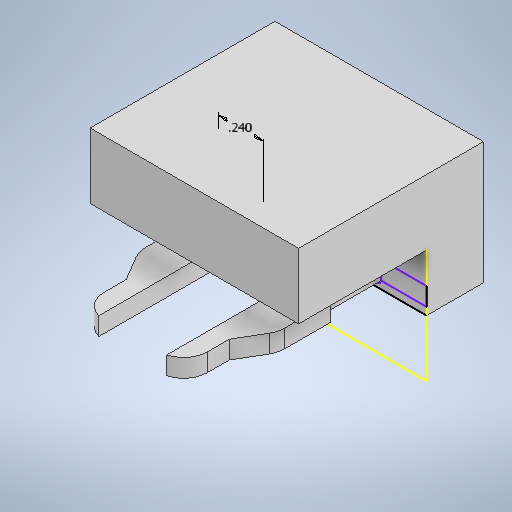
# Autodesk Inventor part: Attachment1
Saved by Autodesk Inventor 2025 (Build 290162010, 162A)
## iProperties
Created: 2026-02-26
Part Number: Attachment1
Material: Generic
Document SubType Name: Modeling
Designer: 925699
Density: 1 g/cm^3
Appearance: Default
Author: 925699
Autodesk Inventor part; units mm, degrees
ref_plane "YZ Plane" through (0, 0, 0) normal (1, 0, 0) x (0, 1, 0)
ref_plane "XZ Plane" through (0, 0, 0) normal (0, 1, 0) x (-1, 0, 0)
ref_plane "XY Plane" through (0, 0, 0) normal (0, 0, 1) x (1, 0, 0)
sketch "Sketch1" plane through (0, 0, 0) normal (0, 0, 1) x (1, 0, 0)
  line L0 (-6.3366, 6.9163) -> (21.6034, 6.9163)
  line L1 (21.6034, 6.9163) -> (21.6034, -8.3237)
  line L2 (21.6034, -8.3237) -> (-6.3366, -8.3237)
  line L3 (-6.3366, -8.3237) -> (-6.3366, 6.9163)
  point P0 (0, 0)
  dimension "d0" = 27.94
  dimension "d1" = 15.24
  constraints: 8 end point, 2 parallel, 1 horizontal, 1 perpendicular
  measures "d0" distance of L1.end L2.end
  measures "d1" distance of L0.end L1.end
extrude "Extrusion1" add sketch "Sketch1" along normal blind 7.62
sketch "Sketch2" plane through (0, 0, 7.62) normal (0, 0, 1) x (1, 0, 0)
  line L0 (-6.3366, 6.9163) -> (-6.3366, -8.3237) projected
  line L1 (21.6034, -8.3237) -> (21.6034, 6.9163) projected
  line L2 (21.6034, 0.3123) -> (21.6034, 2.7253)
  line L3 (-6.3366, 2.7253) -> (-6.3366, 0.3123)
  line L4 (21.6034, 6.9163) -> (-6.3366, 6.9163) projected
  line L5 (-6.3366, -8.3237) -> (21.6034, -8.3237) projected
  line L6 (0.9631, 2.7253) -> (-0.2406, 2.7253)
  line L7 (-0.2406, 0.3123) -> (0.9631, 0.3123)
  line L8 (-0.2406, 0.3123) -> (-0.2406, 2.7253)
  line L9 (-0.2406, 0.3123) -> (3.0821, 0.3123)
  line L10 (3.0821, 0.3123) -> (3.0821, 2.7253)
  line L11 (3.0821, 2.7253) -> (-0.2406, 2.7253)
  line L12 (-0.2406, 2.7253) -> (-0.2406, 0.3123)
  line L13 (14.3038, 2.7253) -> (15.5074, 2.7253)
  line L14 (15.5074, 0.3123) -> (14.3038, 0.3123)
  line L15 (15.5074, 0.3123) -> (15.5074, 2.7253)
  line L16 (15.5074, 0.3123) -> (12.1847, 0.3123)
  line L17 (12.1847, 0.3123) -> (12.1847, 2.7253)
  line L18 (12.1847, 2.7253) -> (15.5074, 2.7253)
  line L19 (15.5074, 2.7253) -> (15.5074, 0.3123)
  line L20 (-6.3366, -0.7037) -> (21.6034, -0.7037)
  line L21 (-6.3366, 2.7253) -> (21.6034, 2.7253)
  line L22 (21.6034, 2.7253) -> (21.6034, 0.3123)
  line L23 (21.6034, 0.3123) -> (-6.3366, 0.3123)
  line L24 (-6.3366, 0.3123) -> (-6.3366, 2.7253)
  point P0 (0, 0)
  point P1 (-0.2406, 1.5188)
  point P2 (15.2669, 0)
  point P3 (15.5074, 1.5188)
  dimension "d6" = 6.096
  constraints: 42 end point, 6 parallel, 4 perpendicular, 3 horizontal, 3 midpoint, 2 point on line
  measures "d6" distance from line of point (-0.241, 1.519) L0
extrude "Extrusion2" add sketch "Sketch2" along normal blind 8.7376 contours L6 L11 L10 L9 L7 L8 | L15 L14 L16 L17 L18 L13
sketch "Sketch3" plane through (-0.2406, 2.7253, 7.62) normal (0, 1, 0) x (1, 0, 0)
  line L0 (3.3227, -8.7376) -> (0, -8.7376) projected
  line L1 (3.3227, -8.7376) -> (0, -8.7376)
  line L2 (-6.096, 7.62) -> (21.844, 7.62) projected
  line L3 (3.3227, -11.3552) -> (3.3227, -8.7376)
  line L4 (12.4253, -8.7376) -> (15.748, -8.7376)
  line L5 (12.4253, -8.7376) -> (15.748, -8.7376)
  line L6 (12.4253, -11.3552) -> (12.4253, -8.7376)
  line L7 (15.748, -8.7376) -> (17.2091, -8.255)
  line L8 (17.2091, -8.255) -> (17.2091, -15.2732)
  line L9 (17.2091, -15.2732) -> (14.9854, -19.057)
  line L10 (14.9854, -19.057) -> (12.4253, -19.057)
  line L11 (12.4253, -19.057) -> (12.4253, -8.7376)
  line L12 (7.874, 7.62) -> (7.874, -24.8322)
  line L13 (3.3227, -8.7376) -> (0, -8.7376)
  line L14 (3.3227, -8.7376) -> (0, -8.7376)
  line L15 (3.3227, -11.3552) -> (3.3227, -8.7376)
  line L16 (0, -8.7376) -> (-1.4611, -8.255)
  line L17 (-1.4611, -8.255) -> (-1.4611, -15.2732)
  line L18 (-1.4611, -15.2732) -> (0.7626, -19.057)
  line L19 (0.7626, -19.057) -> (3.3227, -19.057)
  line L20 (3.3227, -19.057) -> (3.3227, -8.7376)
  point P0 (0.2406, 7.62)
  constraints: 38 end point, 4 symmetric about line, 3 vertical, 2 collinear, 1 midpoint, 1 perpendicular
extrude "Extrusion4" add sketch "Sketch2" along normal blind 25.4 contours L6 L11 L10 L9 L7 L8 | L15 L14 L16 L17 L18 L13
sketch "Sketch4" plane through (-6.3366, 6.9163, 0) normal (0, 1, 0) x (1, 0, 0)
  point P0 (6.3366, 0)
sketch "Sketch5" plane through (0, 0, 7.62) normal (0, 0, 1) x (1, 0, 0)
  line L0 (21.6034, 6.9163) -> (-6.3366, 6.9163) projected
  line L1 (-6.3366, 15.6735) -> (21.6034, 15.6735)
  line L2 (21.6034, 15.6735) -> (21.6034, 6.9163)
  line L3 (21.6034, 6.9163) -> (-6.3366, 6.9163)
  line L4 (-6.3366, 6.9163) -> (-6.3366, 15.6735)
  point P0 (0, 0)
  constraints: 8 end point, 2 parallel, 1 horizontal, 1 perpendicular
extrude "Extrusion5" add sketch "Sketch5" along normal blind 17.145 and the other way blind 7.62
extrude "Extrusion6" cut sketch "Sketch2" against normal blind 25.4 contours L20 L1 L5 L0
extrude "Extrusion7" add sketch "Sketch2" along normal blind 4.7625 contours L21 L8 L23 L0 | L1 L23 L15 L21 | L21 L17 L23 L10
extrude "Extrusion8" add sketch "Sketch3" against normal up to surface (2.413 mm away)
sketch "Sketch6" plane through (-6.3366, 0.3123, 7.62) normal (0, -1, 0) x (1, 0, 0)
  line L0 (27.94, 0) -> (27.94, 4.7625) projected
  line L1 (21.844, 4.7625) -> (21.844, 8.7376) projected
  line L2 (27.94, 0) -> (21.844, 0)
  line L3 (21.844, 0) -> (21.844, 4.7625)
  line L4 (21.844, 4.7625) -> (27.94, 4.7625)
  line L5 (27.94, 4.7625) -> (27.94, 0)
  line L6 (18.5213, 4.7625) -> (18.5213, 25.4) projected
  line L7 (18.5213, 4.7625) -> (9.4187, 4.7625)
  line L8 (9.4187, 4.7625) -> (9.4187, 0)
  line L9 (9.4187, 0) -> (18.5213, 0)
  line L10 (18.5213, 0) -> (18.5213, 4.7625)
  line L11 (6.096, 4.7625) -> (6.096, 8.7376) projected
  line L12 (0, 0) -> (0, 4.7625) projected
  line L13 (6.096, 4.7625) -> (0, 4.7625)
  line L14 (0, 4.7625) -> (0, 0)
  line L15 (0, 0) -> (6.096, 0)
  line L16 (6.096, 0) -> (6.096, 4.7625)
  point P0 (6.3366, -7.62)
  point P1 (18.5213, 19.057)
  constraints: 24 end point, 6 parallel, 3 horizontal, 3 perpendicular, 1 point on line
extrude "Extrusion9" cut sketch "Sketch6" against normal up to surface (6.604 mm away)
sketch "Sketch7" plane through (12.1847, 0.3123, 7.62) normal (0, -1, 0) x (1, 0, 0)
  line L0 (3.3227, 17.7594) -> (4.7838, 15.2732) projected
  line L1 (3.3227, 17.7594) -> (2.3659, 19.3874)
  line L2 (2.3659, 19.3874) -> (2.3659, 25.4)
  line L3 (3.3227, 25.4) -> (0, 25.4) projected
  line L4 (3.3227, 17.7594) -> (3.3227, 25.4) projected
  line L5 (2.3659, 25.4) -> (3.3227, 25.4)
  line L6 (3.3227, 25.4) -> (3.3227, 17.7594)
  line L7 (-18.5213, -7.62) -> (9.4187, -7.62) projected
  line L8 (-12.4253, 17.7594) -> (-11.4685, 19.3874)
  line L9 (-11.4685, 19.3874) -> (-11.4685, 25.4)
  line L10 (-12.4253, 17.7594) -> (-12.4253, 25.4)
  line L11 (-11.4685, 25.4) -> (-12.4253, 25.4)
  line L12 (-12.4253, 25.4) -> (-12.4253, 17.7594)
  point P0 (-12.1847, -7.62)
  constraints: 18 end point, 3 point on line, 2 collinear, 1 horizontal, 1 vertical
extrude "Extrusion10" cut sketch "Sketch7" against normal up to surface (6.604 mm away)
fillet "Fillet1" radius 3.175 4 edges at (0.7162, 1.5188, 33.02) (14.5507, 1.5188, 33.02) (16.9686, 1.5188, 22.8932) (-1.7017, 1.5188, 22.8932)
body "Solid1"
